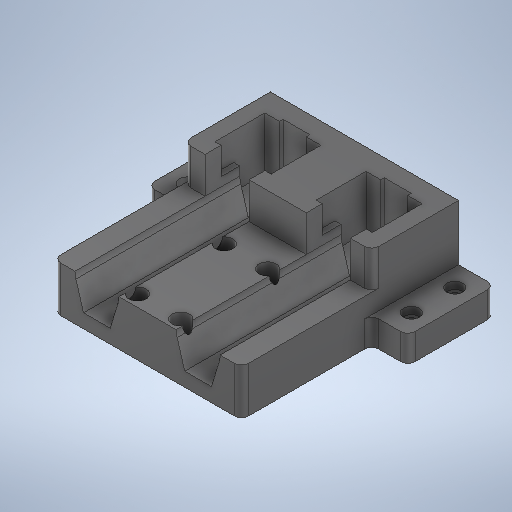
# Autodesk Inventor part: Linear Motor Rear Braket
Saved by Autodesk Inventor 2026.2 (Build 302298010, 298A)
## iProperties
Created: 2026-04-12
Part Number: Linear Motor Rear Braket
Material: ABS Plastic
Document SubType Name: Modeling
Designer: chanh
Density: 1.06 g/cm^3
Appearance: Smooth - White
Author: chanh
Autodesk Inventor part; units mm, degrees
sketch "Sketch1" plane through (0, 0, 0) normal (0, 1, 0) x (-1, 0, 0)
  line L0 (65, -75) -> (-65, -75)
  line L1 (-65, -75) -> (-65, 75)
  line L2 (-65, 75) -> (65, 75)
  line L3 (65, 75) -> (65, -75)
  line L4 (65, -75) -> (-65, 75) construction
  line L5 (-65, -75) -> (65, 75) construction
  point P0 (0, 0)
  dimension "d0" = 130
  dimension "d1" = 150
  constraints: 12 end point, 2 midpoint, 2 parallel, 1 horizontal, 1 perpendicular
  measures "d0" distance of L1.end L2.end
  measures "d1" distance of L0.end L1.end
extrude "Extrusion1" add sketch "Sketch1" along normal blind 31.5
ref_plane "Work Plane6" through (57, 0, -75) normal (0, 0, -1) x (-1, 0, 0)
sketch "Sketch2" plane through (57, 0, -75) normal (0, 0, -1) x (-1, 0, 0)
  circle A0 centre (22, 31.5) radius 10 projected
  line L0 (13, 10) -> (31, 10) projected
  line L1 (31, 10) -> (36.1755, 27.246) projected
  arc A1 (36.1755, 27.246) -> (7.8245, 27.246) centre (22, 31.5) ccw projected
  line L2 (7.8245, 27.246) -> (13, 10) projected
  circle A2 centre (92, 31.5) radius 10 projected
  line L3 (83, 10) -> (101, 10) projected
  line L4 (101, 10) -> (106.1755, 27.246) projected
  arc A3 (106.1755, 27.246) -> (77.8245, 27.246) centre (92, 31.5) ccw projected
  line L5 (77.8245, 27.246) -> (83, 10) projected
  line L6 (36.5586, 27.131) -> (31.2976, 9.6)
  line L7 (31.2976, 9.6) -> (12.7024, 9.6)
  line L8 (12.7024, 9.6) -> (7.4414, 27.131)
  arc A4 (36.5586, 27.131) -> (7.4414, 27.131) centre (22, 31.5) ccw
  line L9 (106.5586, 27.131) -> (101.2976, 9.6)
  line L10 (101.2976, 9.6) -> (82.7024, 9.6)
  line L11 (82.7024, 9.6) -> (77.4414, 27.131)
  arc A5 (106.5586, 27.131) -> (77.4414, 27.131) centre (92, 31.5) ccw
  point P0 (57, 0)
  dimension "d5" = 0.4
  dimension "d6" = 0.4
  constraints: 12 end point, 4 point on circle, 2 centre point, 6 other
  measures "d5" distance between parallel lines of L1 L6
  measures "d6" distance between parallel lines of L4 L9
ref_plane "Work Plane1" through (16, 20, -7.5) normal (0, 0, -1) x (0, 1, 0)
ref_plane "Work Plane3" through (-54, 10, 39) normal (0, 0, -1) x (0, 1, 0)
extrude "Extrusion2" cut sketch "Sketch2" against normal up to surface (114 mm away) contours A0 | L2 A1 L1 L0 | A2 | L5 A3 L4 L3 | L6 L7 L8 A4 | L9 L10 L11 A5
sketch "Sketch3" plane through (50.2, 31.5, 39) normal (0, 0, -1) x (-1, 0, 0)
  arc A0 (-3.8, 34.5) -> (34.2, 34.5) centre (15.2, 34.5) ccw projected
  line L0 (-3.8, 34.5) -> (-3.8, -11.5) projected
  line L1 (-3.8, -11.5) -> (6.2, -21.5) projected
  line L2 (6.2, -21.5) -> (1.0245, -4.254) projected
  arc A1 (29.3755, -4.254) -> (1.0245, -4.254) centre (15.2, 0) ccw projected
  line L3 (29.3755, -4.254) -> (24.2, -21.5) projected
  line L4 (24.2, -21.5) -> (34.2, -11.5) projected
  line L5 (34.2, -11.5) -> (34.2, 34.5) projected
  arc A2 (66.2, 34.5) -> (104.2, 34.5) centre (85.2, 34.5) ccw projected
  line L6 (66.2, 34.5) -> (66.2, -11.5) projected
  line L7 (66.2, -11.5) -> (76.2, -21.5) projected
  line L8 (76.2, -21.5) -> (71.0245, -4.254) projected
  arc A3 (99.3755, -4.254) -> (71.0245, -4.254) centre (85.2, 0) ccw projected
  line L9 (99.3755, -4.254) -> (94.2, -21.5) projected
  line L10 (94.2, -21.5) -> (104.2, -11.5) projected
  line L11 (104.2, -11.5) -> (104.2, 34.5) projected
  line L12 (6.2, -21.5) -> (24.2, -21.5)
  line L13 (-4.2, 8.5) -> (-4.2, -11.5)
  line L14 (-4.2, -11.5) -> (5.8, -21.5)
  line L15 (5.8, -21.5) -> (6.2, -21.5)
  line L16 (-4.2, 8.5) -> (34.6, 8.5)
  line L17 (34.6, 8.5) -> (34.6, -11.5)
  line L18 (34.6, -11.5) -> (24.6, -21.5)
  line L19 (24.6, -21.5) -> (24.2, -21.5)
  line L20 (76.2, -21.5) -> (75.8, -21.5)
  line L21 (75.8, -21.5) -> (65.8, -11.5)
  line L22 (65.8, -11.5) -> (65.8, 8.5)
  line L23 (65.8, 8.5) -> (104.6, 8.5)
  line L24 (104.6, 8.5) -> (104.6, -11.5)
  line L25 (104.6, -11.5) -> (94.6, -21.5)
  line L26 (94.6, -21.5) -> (94.2, -21.5)
  line L27 (76.2, -21.5) -> (94.2, -21.5)
  line L28 (5.8, -21.5) -> (6.2, -21.9)
  line L29 (6.2, -21.9) -> (24.2, -21.9)
  line L30 (24.2, -21.9) -> (24.6, -21.5)
  line L31 (75.8, -21.5) -> (76.2, -21.9)
  line L32 (76.2, -21.9) -> (94.2, -21.9)
  line L33 (94.2, -21.9) -> (94.6, -21.5)
  point P0 (50.1, -31.5)
  point P1 (104.2, 8.5)
  point P2 (66.2, 8.5)
  point P3 (-3.8, 8.5)
  point P4 (34.2, 8.5)
  dimension "d9" = 0.4
  dimension "d10" = 0.4
  dimension "d11" = 0.4
  dimension "d12" = 0.4
  dimension "d13" = 30
  dimension "d14" = 0.4
  dimension "d53" = 0.4
  dimension "d54" = 0.4
  constraints: 44 end point, 9 collinear, 5 horizontal, 4 horizontal alignment, 4 perpendicular, 3 parallel, 1 point on line, 1 vertical
  measures "d9" distance of L14.end L1.end
  measures "d10" distance between parallel lines of L0 L13
  measures "d11" distance of L18.end L3.end
  measures "d12" distance between parallel lines of L5 L17
  measures "d13" distance between parallel lines of L16 L12
  measures "d14" distance of L7.end L20.end
  measures "d53" distance between parallel lines of L12 L29
  measures "d54" distance between parallel lines of L27 L32
extrude "Extrusion7" cut sketch "Sketch3" against normal blind 21.5
sketch "Sketch8" plane through (0, 31.5, 0) normal (0, 1, 0) x (1, 0, 0)
  line L0 (65, -75) -> (65, 75) projected
  line L1 (-65, 75) -> (-65, -75) projected
  line L2 (0, 75) -> (0, -65) construction
  line L3 (-65, -75) -> (65, -75) projected
  line L4 (-50.2, 75) -> (-65, 75) projected
  line L5 (-50.2, -39) -> (-50.2, 75) projected
  line L6 (65, 75) -> (50.2, 75) projected
  line L7 (50.2, 75) -> (50.2, -39) projected
  line L8 (19.8, -39) -> (19.8, 75) projected
  line L9 (19.8, 75) -> (-19.8, 75) projected
  line L10 (-19.8, 75) -> (-19.8, -39) projected
  line L11 (-19.8, -39) -> (-15.6, -39) projected
  line L12 (-15.6, -39) -> (-15.6, -60.5) projected
  line L13 (-15.6, -60.5) -> (-54.4, -60.5) projected
  line L14 (-54.4, -60.5) -> (-54.4, -39) projected
  line L15 (-54.4, -39) -> (-50.2, -39) projected
  line L16 (50.2, -39) -> (54.4, -39) projected
  line L17 (54.4, -39) -> (54.4, -60.5) projected
  line L18 (54.4, -60.5) -> (15.6, -60.5) projected
  line L19 (15.6, -60.5) -> (15.6, -39) projected
  line L20 (15.6, -39) -> (19.8, -39) projected
  point P0 (0, 0)
  point P1 (-15, 67)
  point P2 (-15, 7)
  point P3 (15, 67)
  point P4 (15, 7)
  dimension "d31" = 15
  dimension "d32" = 60
  constraints: 2 end point, 2 symmetric about line, 1 vertical alignment
  measures "d31" distance from line of point (-15, 67) L2
  measures "d32" distance of point (-15, 67) point (-15, 7)
hole "Hole2" at (-15, 31.5, -67) at (-15, 31.5, -7) at (15, 31.5, -7) at (15, 31.5, -67) direction (0, -1, 0) diameter 6.2 end through all counterbore diameter 12 counterbore depth 18.5
sketch "Sketch9" plane through (0, 0, 0) normal (0, -1, 0) x (1, 0, 0)
  circle A0 centre (-35, 32) radius 1.621 projected
  circle A1 centre (35, 32) radius 1.621 projected
  point P0 (0, 0)
hole "Hole3" at (-35, 0, 32) at (35, 0, 32) direction (0, 1, 0) diameter 4.2 end through all counterbore diameter 10 counterbore depth 3.7
sketch "Sketch12" plane through (0, 31.5, 0) normal (0, 1, 0) x (1, 0, 0)
  arc A0 (19.8, 70.6) -> (19.8, 63.4) centre (15, 67) ccw projected
  line L0 (19.8, 70.6) -> (19.8, 75) projected
  line L1 (19.8, 75) -> (-19.8, 75) projected
  line L2 (-19.8, 75) -> (-19.8, 70.6) projected
  arc A1 (-19.8, 63.4) -> (-19.8, 70.6) centre (-15, 67) ccw projected
  line L3 (-19.8, 63.4) -> (-19.8, 10.6) projected
  arc A2 (-19.8, 3.4) -> (-19.8, 10.6) centre (-15, 7) ccw projected
  line L4 (-19.8, 3.4) -> (-19.8, -39) projected
  line L5 (-19.8, -39) -> (-15.6, -39) projected
  line L6 (-15.6, -39) -> (-15.6, -60.5) projected
  line L7 (-15.6, -60.5) -> (-54.4, -60.5) projected
  line L8 (-54.4, -60.5) -> (-54.4, -39) projected
  line L9 (-54.4, -39) -> (-50.2, -39) projected
  line L10 (-50.2, -39) -> (-50.2, 75) projected
  line L11 (-50.2, 75) -> (-65, 75) projected
  line L12 (-65, 75) -> (-65, -75) projected
  line L13 (-65, -75) -> (65, -75) projected
  line L14 (65, -75) -> (65, 75) projected
  line L15 (65, 75) -> (50.2, 75) projected
  line L16 (50.2, 75) -> (50.2, -39) projected
  line L17 (50.2, -39) -> (54.4, -39) projected
  line L18 (54.4, -39) -> (54.4, -60.5) projected
  line L19 (54.4, -60.5) -> (15.6, -60.5) projected
  line L20 (15.6, -60.5) -> (15.6, -39) projected
  line L21 (15.6, -39) -> (19.8, -39) projected
  line L22 (19.8, -39) -> (19.8, 3.4) projected
  arc A3 (19.8, 10.6) -> (19.8, 3.4) centre (15, 7) ccw projected
  line L23 (19.8, 10.6) -> (19.8, 63.4) projected
  line L24 (65, -15) -> (-65, -15)
  point P0 (0, 0)
  point P1 (-50.2, -15)
  point P2 (50.2, -15)
  point P3 (19.8, -15)
  point P4 (-19.8, -15)
  dimension "d55" = 60
  constraints: 2 end point, 2 point on line, 1 horizontal
  measures "d55" distance between parallel lines of L13 L24
extrude "Extrusion8" add sketch "Sketch12" along normal blind 25 contours L22 L21 L20 L19 L18 L17 L16 L24 L14 L13 L12 L10 L9 L8 L7 L6 L5 L4
sketch "Sketch13" plane through (50.2, 31.5, 60.5) normal (0, 0, -1) x (-1, 0, 0)
  line L0 (-4.2, -11.5) -> (-4.2, 25) projected
  line L1 (6.2, -21.9) -> (-4.2, -11.5) projected
  line L2 (24.2, -21.9) -> (6.2, -21.9) projected
  line L3 (34.6, -11.5) -> (24.2, -21.9) projected
  line L4 (34.6, 25) -> (34.6, -11.5) projected
  line L5 (-4.2, 25) -> (34.6, 25) projected
  line L6 (65.8, -11.5) -> (65.8, 25) projected
  line L7 (76.2, -21.9) -> (65.8, -11.5) projected
  line L8 (94.2, -21.9) -> (76.2, -21.9) projected
  line L9 (104.6, -11.5) -> (94.2, -21.9) projected
  line L10 (104.6, 25) -> (104.6, -11.5) projected
  line L11 (65.8, 25) -> (104.6, 25) projected
  line L12 (5.95, 25) -> (24.45, 25)
  line L13 (24.45, 25) -> (24.45, -10.9)
  line L14 (24.45, -10.9) -> (5.95, -10.9)
  line L15 (5.95, -10.9) -> (5.95, 25)
  line L16 (5.95, 25) -> (24.45, -10.9) construction
  line L17 (24.45, 25) -> (5.95, -10.9) construction
  line L18 (50.2, -31.5) -> (50.2, 25) construction
  line L19 (94.45, 25) -> (75.95, 25)
  line L20 (75.95, 25) -> (75.95, -10.9)
  line L21 (75.95, -10.9) -> (94.45, -10.9)
  line L22 (94.45, -10.9) -> (94.45, 25)
  line L23 (94.45, 25) -> (75.95, -10.9) construction
  line L24 (75.95, 25) -> (94.45, -10.9) construction
  point P0 (15.2, 7.05)
  point P1 (15.2, -21.9)
  point P2 (15.2, 25)
  point P3 (85.2, 7.05)
  point P4 (85.2, 25)
  point P5 (75.95, 25)
  point P6 (24.45, 25)
  point P7 (5.95, 25)
  dimension "d58" = 18.5
  dimension "d59" = 11
  constraints: 26 end point, 6 symmetric about line, 5 midpoint, 2 parallel, 1 horizontal, 1 perpendicular, 1 vertical, 1 vertical alignment
  measures "d58" distance of L12.start L12.end
  measures "d59" distance between parallel lines of L2 L14
extrude "Extrusion9" cut sketch "Sketch13" against normal blind 2.5 contours L5 L13 L14 L15 | L11 L22 L21 L20
sketch "Sketch14" plane through (65, 0, 75) normal (1, 0, 0) x (0, 0, -1)
  line L0 (0, 0) -> (150, 0) projected
  line L1 (150, 0) -> (150, 31.5) projected
  line L2 (60, 31.5) -> (150, 31.5) projected
  line L3 (60, 31.5) -> (60, 56.5) projected
  line L4 (0, 56.5) -> (60, 56.5) projected
  line L5 (0, 0) -> (0, 56.5) projected
  line L6 (0, 0) -> (60, 0)
  line L7 (60, 0) -> (60, 18)
  line L8 (60, 18) -> (0, 18)
  line L9 (0, 18) -> (0, 0)
  point P0 (75, 0)
  dimension "d62" = 60
  dimension "d63" = 18
  constraints: 8 end point, 2 parallel, 1 horizontal, 1 perpendicular
  measures "d62" distance of L8.end L7.end
  measures "d63" distance of L7.end L6.end
extrude "Extrusion10" add sketch "Sketch14" along normal blind 25 contours L5 L8 L7 L0
sketch "Sketch15" plane through (65, 18, 75) normal (0, 1, 0) x (1, 0, 0)
  line L0 (0, 0) -> (0, 60) projected
  line L1 (0, 0) -> (25, 0) projected
  line L2 (25, 60) -> (25, 0) projected
  line L3 (0, 60) -> (25, 60) projected
  line L4 (25, 30) -> (0, 30) construction
  point P0 (-65, 75)
  point P1 (12.5, 15)
  point P2 (12.5, 45)
  point P3 (12.5, 0)
  dimension "d66" = 30
  constraints: 3 midpoint, 2 end point, 2 vertical alignment, 1 symmetric about line
  measures "d66" distance of point (12.5, 45) point (12.5, 15)
hole "Hole4" at (77.5, 18, 60) at (77.5, 18, 30) direction (0, -1, 0) diameter 6.2 end through all counterbore diameter 11 counterbore depth 5
mirror "Mirror1" about plane through (0, 0, 0) normal (1, 0, 0) of "Hole4", "Extrusion10"
fillet "Fillet4" radius 5 10 edges at (-65, 15.75, -75) (65, 15.75, -75) (-65, 9, 15) (-90, 9, 15) (-90, 9, 75) (90, 9, 75) (90, 9, 15) (65, 9, 15) (65, 44, 15) (-65, 44, 15)
sketch "Sketch16" plane through (0, 56.5, 0) normal (0, 1, 0) x (1, 0, 0)
  arc A0 (-60, -15) -> (-65, -20) centre (-60, -20) ccw projected
  line L0 (-65, -20) -> (-65, -75) projected
  line L1 (-65, -75) -> (65, -75) projected
  line L2 (65, -75) -> (65, -20) projected
  arc A1 (65, -20) -> (60, -15) centre (60, -20) ccw projected
  line L3 (60, -15) -> (50.2, -15) projected
  line L4 (50.2, -15) -> (50.2, -39) projected
  line L5 (50.2, -39) -> (54.4, -39) projected
  line L6 (54.4, -39) -> (54.4, -60.5) projected
  line L7 (54.4, -60.5) -> (44.25, -60.5) projected
  line L8 (44.25, -60.5) -> (44.25, -63) projected
  line L9 (44.25, -63) -> (25.75, -63) projected
  line L10 (25.75, -63) -> (25.75, -60.5) projected
  line L11 (25.75, -60.5) -> (15.6, -60.5) projected
  line L12 (15.6, -60.5) -> (15.6, -39) projected
  line L13 (15.6, -39) -> (19.8, -39) projected
  line L14 (19.8, -39) -> (19.8, -15) projected
  line L15 (19.8, -15) -> (-19.8, -15) projected
  line L16 (-19.8, -15) -> (-19.8, -39) projected
  line L17 (-19.8, -39) -> (-15.6, -39) projected
  line L18 (-15.6, -39) -> (-15.6, -60.5) projected
  line L19 (-15.6, -60.5) -> (-25.75, -60.5) projected
  line L20 (-25.75, -60.5) -> (-25.75, -63) projected
  line L21 (-25.75, -63) -> (-44.25, -63) projected
  line L22 (-44.25, -63) -> (-44.25, -60.5) projected
  line L23 (-44.25, -60.5) -> (-54.4, -60.5) projected
  line L24 (-54.4, -60.5) -> (-54.4, -39) projected
  line L25 (-54.4, -39) -> (-50.2, -39) projected
  line L26 (-50.2, -39) -> (-50.2, -15) projected
  line L27 (-50.2, -15) -> (-60, -15) projected
  line L28 (50.2, -39) -> (54.4, -39)
  line L29 (54.4, -39) -> (54.4, -26)
  line L30 (54.4, -26) -> (50.2, -26)
  line L31 (50.2, -26) -> (50.2, -39)
  line L32 (54.4, -39) -> (54.4, -60.5) projected
  line L33 (19.8, -39) -> (15.6, -39)
  line L34 (15.6, -39) -> (15.6, -26)
  line L35 (15.6, -26) -> (19.8, -26)
  line L36 (19.8, -26) -> (19.8, -39)
  line L37 (15.6, -60.5) -> (15.6, -39) projected
  line L38 (0, -75) -> (0, -15) construction
  line L39 (-50.2, -39) -> (-54.4, -39)
  line L40 (-15.6, -39) -> (-19.8, -39)
  line L41 (-50.2, -39) -> (-54.4, -39)
  line L42 (-54.4, -39) -> (-54.4, -26)
  line L43 (-54.4, -26) -> (-50.2, -26)
  line L44 (-50.2, -26) -> (-50.2, -39)
  line L45 (-19.8, -39) -> (-15.6, -39)
  line L46 (-15.6, -39) -> (-15.6, -26)
  line L47 (-15.6, -26) -> (-19.8, -26)
  line L48 (-19.8, -26) -> (-19.8, -39)
  point P0 (0, 0)
  dimension "d75" = 13
  constraints: 38 end point, 8 symmetric about line, 4 parallel, 3 collinear, 2 horizontal, 2 midpoint, 2 perpendicular
  measures "d75" distance of L29.end L28.end
extrude "Extrusion11" cut sketch "Sketch16" against normal blind 18.9 contours L26 L25 L42 L43 | L30 L29 L5 L4 | L17 L16 L47 L46 | L34 L35 L14 L13
equation "\"d10\" = d9"
equation "\"d11\" = d9"
equation "\"d12\" = d9"
equation "\"d14\" = d9"
equation "\"d53\" = d9"
equation "\"d54\" = d9"
body "Solid1"
